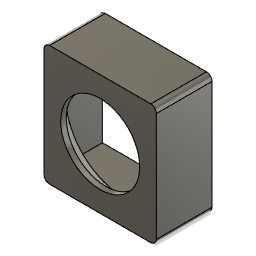
nebula_adapter (Autodesk Fusion 360 design; units mm, degrees)
Autodesk Fusion 360 part; units mm, degrees
sketch "Skizze1" plane through (0, 0, 0) normal (0, 0, 1) x (1, 0, 0)
  circle A0 centre (0, 0) radius 7.1
  line L0 (10.1, 10.8) -> (-10.1, 10.8)
  line L1 (-10.1, 10.8) -> (-10.1, -10.8)
  line L2 (-10.1, -10.8) -> (10.1, -10.8)
  line L3 (10.1, -10.8) -> (10.1, 10.8)
  line L4 (10.1, 10.8) -> (-10.1, -10.8) construction
  line L5 (-10.1, 10.8) -> (10.1, -10.8) construction
  dimension "d1" = 14.2
  dimension "d2" = 20.2
  dimension "d3" = 21.6
  constraint coincident A0.centre origin
  constraint horizontal L0
  constraint perpendicular L0 L1
  constraint parallel L0 L2
  constraint parallel L1 L3
  constraint coincident L4 A0.centre
  constraint coincident L5 A0.centre
  measures "d1" diameter of A0
  measures "d2" distance of L1.end L2.end
  measures "d3" distance of L0.end L1.end
extrude "Extrusion1" add sketch "Skizze1" against normal blind 10
sketch "Skizze2" plane through (0, 0, -10) normal (0, 0, -1) x (-1, 0, 0)
  circle A0 centre (0, 0) radius 7.1
  line L0 (-10.1, 10.8) -> (-10.1, -10.8)
  line L1 (-10.1, -10.8) -> (10.1, -10.8)
  line L2 (10.1, -10.8) -> (10.1, 10.8)
  line L3 (10.1, 10.8) -> (-10.1, 10.8)
  line L4 (9.6, 9.6) -> (-9.6, 9.6)
  line L5 (-9.6, 9.6) -> (-9.6, -9.6)
  line L6 (-9.6, -9.6) -> (9.6, -9.6)
  line L7 (9.6, -9.6) -> (9.6, 9.6)
  line L8 (9.6, 9.6) -> (-9.6, -9.6) construction
  line L9 (-9.6, 9.6) -> (9.6, -9.6) construction
  dimension "d6" = 19.2
  dimension "d7" = 19.2
  constraint horizontal L4
  constraint perpendicular L4 L5
  constraint parallel L4 L6
  constraint parallel L5 L7
  constraint coincident L8 A0.centre
  constraint coincident L9 A0.centre
  constraint coincident A0.centre origin
  measures "d6" distance of L5.end L6.end
  measures "d7" distance of L4.end L5.end
extrude "Extrusion2" cut sketch "Skizze2" against normal blind 6 contours L4 L5 L6 L7
chamfer "Fase1" distance 3 angle 45 1 edges at (-6.6195, 2.5675, -4)
fillet "Abrundung1" radius 1 4 edges at (-10.1, 10.8, -5) (10.1, 10.8, -5) (-10.1, -10.8, -5) (10.1, -10.8, -5)
equation "d6 = d7"
